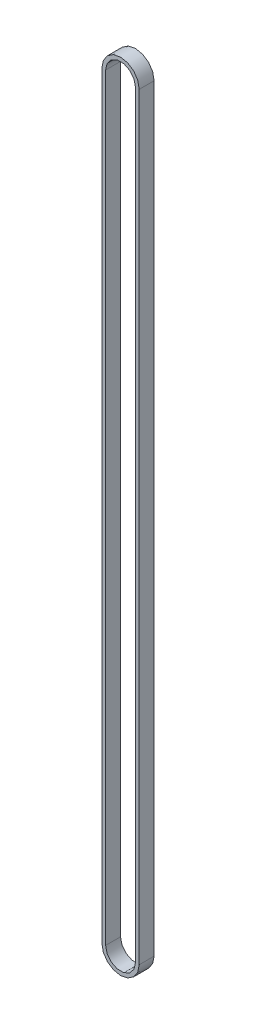
# Autodesk Inventor part: Y belt
Saved by Autodesk Inventor 2017 (Build 210142000, 142)
## iProperties
Part Number: Y belt
Material: Gummi, Silikon
Document SubType Name: Modeling
Designer: Till
Density: 1.25 g/cm^3
Appearance: Gummi - schwarz
Author: Till
Autodesk Inventor part; units mm, degrees
ref_plane "YZ Plane" through (0, 0, 0) normal (1, 0, 0) x (0, 1, 0)
ref_plane "XZ Plane" through (0, 0, 0) normal (0, 1, 0) x (-1, 0, 0)
ref_plane "XY Plane" through (0, 0, 0) normal (0, 0, 1) x (1, 0, 0)
sketch "Skizze1" plane through (0, 0, 0) normal (0, 0, 1) x (1, 0, 0)
  arc A0 (6, 0) -> (-6, 0) centre (0, 0) ccw
  arc A1 (7.5, 0) -> (-7.5, 0) centre (0, 0) ccw
  arc A2 (-6, -305.0274) -> (6, -305.0274) centre (0, -305.0274) ccw
  line L0 (0, -305.0274) -> (6, -305.0274) construction
  line L1 (0, -305.0274) -> (-6, -305.0274) construction
  arc A3 (-7.5, -305.0274) -> (7.5, -305.0274) centre (0, -305.0274) ccw
  line L2 (0, -305.0274) -> (7.5, -305.0274) construction
  line L3 (0, -305.0274) -> (-7.5, -305.0274) construction
  line L4 (-7.5, -305.0274) -> (-7.5, 0)
  line L5 (-6, 0) -> (-6, -305.0274)
  line L6 (6, -305.0274) -> (6, 0)
  line L7 (7.5, -305.0274) -> (7.5, 0)
  dimension "d0" = 6
  dimension "d1" = 7.5
  dimension "d2" = 6
  dimension "d3" = 180
  dimension "d4" = 7.5
  dimension "d5" = 180
  dimension "d6" = 305.0274
  dimension "d7" = 0
  constraints: 16 end point, 8 point on circle, 4 centre point, 3 coincident, 3 parallel, 1 tangent, 1 vertical
  measures "d0" radius of A0
  measures "d1" radius of A1
  measures "d2" radius of A2
  measures "d3" angle of L1 L0
  measures "d4" radius of A3
  measures "d5" angle of L3 L2
  measures "d6" distance of point (0, 0) L0.start
  measures "d7" vertical distance of point (0, 0) L6.end
extrude "Extrusion1" add sketch "Skizze1" along normal blind 6
